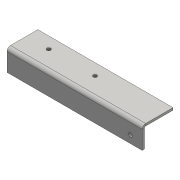
# Autodesk Inventor part: endcapOptionRightAngle
Saved by Autodesk Inventor 2016 (Build 200138000, 138)
## iProperties
Created: 2015-05-26
Part Number: endcapOptionRightAngle
Material: Generic
Document SubType Name: Sheet Metal
Designer: krosie
Density: 1 g/cm^3
Sheet Metal Rule: Copy of Default_mm
Appearance: Default
Flat Pattern Width: 6.34296 cm
Flat Pattern Length: 17.5 cm
Flat Pattern Area: 111.002 cm^2
Sheet Metal Width: 63.430 mm
Sheet Metal Length: 175.000 mm
Sheet Metal Area: 11100.188 mm^2
Author: krosie
Autodesk Inventor part; units mm, degrees
ref_plane "YZ Plane" through (0, 0, 0) normal (1, 0, 0) x (0, 1, 0)
ref_plane "XZ Plane" through (0, 0, 0) normal (0, 1, 0) x (-1, 0, 0)
ref_plane "XY Plane" through (0, 0, 0) normal (0, 0, 1) x (1, 0, 0)
sketch "Sketch1" plane through (0, 0, 0) normal (0, 0, 1) x (1, 0, 0)
  line L0 (0, 0) -> (175, 0)
  line L1 (175, 0) -> (175, 40)
  line L2 (175, 40) -> (0, 40)
  line L3 (0, 40) -> (0, 0)
  dimension "d0" = 175
  dimension "d1" = 40
  measures "d0" distance of L0.start L0.end
  measures "d1" distance of L0.end L1.end
extrude "Plate1" add sketch "Sketch1" along normal blind 3
sketch "Sketch2" plane through (0, 0, 0) normal (0, -1, 0) x (1, 0, 0)
  line L0 (0, 0) -> (0, -25)
  line L1 (0, -25) -> (175, -25)
  line L2 (175, -25) -> (175, 0)
  line L3 (0, 0) -> (175, 0)
  line L4 (175, 0) -> (0, 0)
  dimension "d3" = 25
  dimension "d4" = 175
  measures "d3" distance of L0.start L0.end
  measures "d4" distance of L0.end L1.end
sheet face with bend "Face2" sketch "Sketch2" thickness 3 toward (0, 1, 0) bend radius 1.5 relief straight relief width 3 relief depth 1.5
bend "Bend1"
hole "Hole1" at (29, 25, 0) direction (0, 0, 1) diameter 5 end through all
hole "Hole2" at (89, 25, 0) direction (0, 0, 1) diameter 5 end through all
hole "Hole3" at (160, 3, -15) direction (0, -1, 0) diameter 5 end through all
equation "\"d17\" = Thickness"
equation "\"d26\" = Thickness"
equation "\"d35\" = Thickness"
equation "\"d6\" = BendReliefWidth"
equation "\"d8\" = MinimumRemnant"
equation "\"d7\" = BendReliefDepth"
equation "\"d9\" = BendRadius"
equation "\"BendRadius\" = Thickness"
equation "\"BendReliefWidth\" = Thickness"
equation "\"BendReliefDepth\" = 0.5 * Thickness"
equation "\"CornerReliefSize\" = 4 * Thickness"
equation "\"MinimumRemnant\" = 2 * Thickness"
equation "\"TransitionRadius\" = BendRadius"
equation "\"JacobiRadiusSize\" = BendRadius"
equation "\"GapSize\" = Thickness"
equation "\"d2\" = BendRadius"
equation "\"Thickness\" = 3"
body "Solid1"
